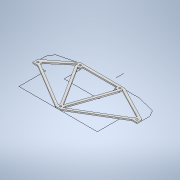
# Autodesk Inventor part: ScrewHoleGuide
Saved by Autodesk Inventor 2020 (Build 240168000, 168)
## iProperties
Created: 2024-02-16
Part Number: ScrewHoleGuide
Material: Generic
Document SubType Name: Modeling
Designer: smz3rm
Density: 1 g/cm^3
Appearance: Default
Author: smz3rm
Autodesk Inventor part; units mm, degrees
ref_plane "YZ Plane" through (0, 0, 0) normal (1, 0, 0) x (0, 1, 0)
ref_plane "XZ Plane" through (0, 0, 0) normal (0, 1, 0) x (-1, 0, 0)
ref_plane "XY Plane" through (0, 0, 0) normal (0, 0, 1) x (1, 0, 0)
sketch "Sketch1" plane through (0, 0, 0) normal (0, 1, 0) x (-1, 0, 0)
  line L0 (8, 0) -> (8, 8) projected
  line L1 (8, 8) -> (0, 8)
  line L2 (0, 8) -> (0, 0)
  line L3 (0, 0) -> (8, 0)
  line L4 (8, 0) -> (8, 8)
  line L5 (49.4, -65) -> (41.4, -65) projected
  line L6 (49.4, -65) -> (41.4, -65)
  line L7 (41.4, -65) -> (41.4, -73)
  line L8 (41.4, -73) -> (49.4, -73)
  line L9 (49.4, -73) -> (49.4, -65)
  line L10 (80, -35.15) -> (80, -43.15) projected
  line L11 (88, -35.15) -> (80, -35.15)
  line L12 (80, -35.15) -> (80, -43.15)
  line L13 (80, -43.15) -> (88, -43.15)
  line L14 (88, -43.15) -> (88, -35.15)
  line L15 (-22.4, -65) -> (-14.4, -65) projected
  line L16 (-22.4, -73) -> (-22.4, -65) projected
  line L17 (-14.4, -65) -> (-22.4, -65)
  line L18 (-22.4, -65) -> (-22.4, -73)
  line L19 (-22.4, -73) -> (-14.4, -73)
  line L20 (-14.4, -73) -> (-14.4, -65)
  line L21 (-72, -43.15) -> (-72, -35.15) projected
  line L22 (-80, -43.15) -> (-72, -43.15) projected
  line L23 (-72, -35.15) -> (-80, -35.15)
  line L24 (-80, -35.15) -> (-80, -43.15)
  line L25 (-80, -43.15) -> (-72, -43.15)
  line L26 (-72, -43.15) -> (-72, -35.15)
  circle A0 centre (-76, -39.15) radius 1.6
  circle A1 centre (-18.4, -69) radius 1.6
  circle A2 centre (45.4, -69) radius 1.6
  circle A3 centre (84, -39.15) radius 1.6
  circle A4 centre (4, 4) radius 1.6
  line L27 (0, 0) -> (8, 0) projected
  line L28 (41.4, -65) -> (41.4, -73) projected
  line L29 (41.4, -73) -> (-14.4, -73)
  line L30 (-80, -43.15) -> (-22.4, -73)
  line L31 (88, -43.15) -> (49.4, -73)
  line L32 (0, 8) -> (0, 0) projected
  line L33 (0, 8) -> (-72, -35.15)
  line L34 (8, 8) -> (80, -35.15)
  line L35 (80, -39.15) -> (8, 4)
  line L36 (0, 4) -> (-72, -39.15)
  line L37 (-22.4, -69) -> (-72.2814, -43.15)
  line L38 (80, -43.15) -> (49.4, -69)
  line L39 (49.4, -73) -> (49.4, -65) projected
  line L40 (41.4, -69) -> (-14.4, -69)
  line L41 (-14.4, -65) -> (-14.4, -73) projected
  line L42 (4, 0) -> (45.4, -65)
  line L43 (8, 0) -> (49.4, -65)
  line L44 (0, 0) -> (-22.4, -65)
  line L45 (-18.4, -65) -> (4, 0)
  point P0 (-14.4, -69)
  dimension "d0" = 3.2
  constraints: 68 end point, 14 parallel, 10 midpoint, 6 perpendicular, 5 centre point, 5 horizontal, 4 equal radius, 1 point on line
  measures "d0" diameter of A0
extrude "Extrusion1" add sketch "Sketch1" along normal blind 2 contours L3 L2 L1 L0 | L43 L5 L42 L3 | L0 L34 L10 L35 | L45 L15 L44 L3 | L9 L8 L7 L5 | L10 L11 L14 L13 | L15 L20 L19 L16 | L38 L13 L31 L9 | L2 L36 L21 L33 | L21 L22 L24 L23 | L16 L30 L22 L37 | L7 L29 L20 L40
body "Solid1"
